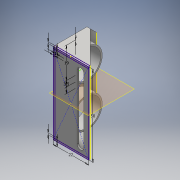
# Autodesk Inventor part: Ultra Sonic Sensor Mounting
Saved by Autodesk Inventor 2016 (Build 200138000, 138)
## iProperties
Created: 2016-05-08
Part Number: Ultra Sonic Sensor Mounting
Material: Generic
Document SubType Name: Modeling
Designer: Kenneth Daniel
Density: 1 g/cm^3
Appearance: Default
Author: Kenneth Daniel
Autodesk Inventor part; units mm, degrees
ref_plane "YZ Plane" through (0, 0, 0) normal (1, 0, 0) x (0, 1, 0)
ref_plane "XZ Plane" through (0, 0, 0) normal (0, 1, 0) x (-1, 0, 0)
ref_plane "XY Plane" through (0, 0, 0) normal (0, 0, 1) x (1, 0, 0)
sketch "Sketch1" plane through (0, 0, 0) normal (0, 1, 0) x (-1, 0, 0)
  line L0 (-11, 25) -> (-11, -25)
  line L1 (-11, -25) -> (11, -25)
  line L2 (11, -25) -> (11, 25)
  line L3 (11, 25) -> (-11, 25)
  line L4 (-11, 25) -> (11, -25) construction
  line L5 (-11, -25) -> (11, 25) construction
  line L6 (11, 25) -> (10, 25)
  line L7 (10, 25) -> (10, -25)
  line L8 (11, 25) -> (11, 24)
  line L9 (11, 24) -> (-11, 24)
  line L10 (11, -25) -> (11, -24)
  line L11 (11, -24) -> (-11, -24)
  point P0 (0, 0)
  dimension "d0" = 50
  dimension "d1" = 22
  dimension "d2" = 1
  dimension "d3" = 1
  dimension "d4" = 1
  constraints: 24 end point, 6 point on line, 4 perpendicular, 2 midpoint, 2 parallel, 1 vertical
  measures "d0" distance of L0.start L0.end
  measures "d1" distance of L1.end L0.end
  measures "d2" distance of L2.end L6.end
  measures "d3" distance of L2.end L8.end
  measures "d4" distance of L1.end L10.end
extrude "Extrusion1" add sketch "Sketch1" along normal blind 1
sketch "Sketch2" plane through (0, 1, 0) normal (0, 1, 0) x (1, 0, 0)
  line L0 (11, -25) -> (11, 25) projected
  line L1 (-11, -25) -> (11, -25) projected
  line L2 (11, -25) -> (-11, -25)
  line L3 (-11, -25) -> (-11, -24)
  line L4 (-11, 25) -> (-11, -25) projected
  line L5 (-11, -24) -> (11, -24)
  line L6 (-11, -25) -> (-10, -25)
  line L7 (-10, -25) -> (-10, 25)
  line L8 (11, 25) -> (-11, 25) projected
  line L9 (-11, 25) -> (-11, 24)
  line L10 (-11, 24) -> (11, 24)
  point P0 (0, 0)
  dimension "d7" = 1
  dimension "d8" = 1
  dimension "d9" = 1
  constraints: 14 end point, 6 point on line, 3 perpendicular, 1 collinear
  measures "d7" distance of L1.start L3.end
  measures "d8" distance of L1.start L6.end
  measures "d9" distance of L4.start L9.end
extrude "Extrusion2" add sketch "Sketch2" along normal blind 25 contours L1 L3 L5 L7 | L5 L4 L10 L7 | L10 L4 L8 L7
extrude "Extrusion3" add sketch "Sketch2" along normal blind 25 contours L1 L7 L5 L0 | L1 L3 L5 L7 | L10 L7 L8 L0 | L10 L4 L8 L7
sketch "Sketch3" plane through (-11, 0, 25) normal (0, 0, 1) x (1, 0, 0)
  point P0 (11, 0)
sketch "Sketch4" plane through (-11, 0, -25) normal (-1, 0, 0) x (0, 0, 1)
  line L0 (49, 26) -> (1, 26) projected
  line L1 (25, 26) -> (45, 26)
  line L2 (25, 26) -> (5, 26)
  line L3 (50, 0) -> (50, 26) projected
  line L4 (50, 26) -> (50, 21)
  line L5 (50, 21) -> (45, 26)
  line L6 (0, 0) -> (0, 26) projected
  line L7 (0, 26) -> (0, 21)
  line L8 (0, 21) -> (5, 26)
  line L9 (50, 26) -> (45, 26)
  line L10 (0, 26) -> (5, 26)
  line L11 (0, 26) -> (50, 26) projected
  point P0 (25, 0)
  dimension "d14" = 20
  dimension "d15" = 20
  dimension "d16" = 5
  dimension "d17" = 5
  constraints: 16 end point, 4 point on line, 2 collinear, 1 midpoint
  measures "d14" distance of L1.start L1.end
  measures "d15" distance of L1.start L2.end
  measures "d16" distance of L3.end L4.end
  measures "d17" distance of L6.end L7.end
extrude "Extrusion4" cut sketch "Sketch4" against normal blind 25
sketch "Sketch5" plane through (-11, 0, 25) normal (0, 0, 1) x (1, 0, 0)
  line L0 (1, 22) -> (1, 26) projected
  line L1 (1, 22) -> (22, 1)
  line L2 (22, 22) -> (1, 22) projected
  line L3 (1, 22) -> (22, 22)
  line L4 (22, 22) -> (22, 1)
  point P0 (11, 0)
  constraints: 6 end point, 1 collinear, 1 perpendicular
extrude "Extrusion5" cut sketch "Sketch5" against normal through all
sketch "Sketch6" plane through (-10, 1, 24) normal (1, 0, 0) x (0, 0, -1)
  line L0 (4, 25) -> (44, 25) projected
  line L1 (24, 25) -> (24, -1) construction
  line L2 (0, 21) -> (0, 0) construction
  line L3 (0, 12) -> (48, 12) construction
  line L4 (48, 0) -> (48, 21) construction
  line L5 (24, 12) -> (20.5, 12) construction
  line L6 (20.5, 12) -> (27.5, 12) construction
  line L7 (20.5, 12) -> (1.5, 12) construction
  circle A0 centre (11, 12) radius 9.5
  circle A1 centre (11, 12) radius 8.5
  dimension "d22" = 3.5
  dimension "d23" = 7
  dimension "d24" = 19
  dimension "d25" = 1
  constraints: 10 end point, 5 point on line, 3 midpoint, 1 centre point, 1 horizontal, 1 horizontal alignment, 1 vertical, 2 other
  measures "d22" distance of L5.start L5.end
  measures "d23" distance of L5.end L6.end
  measures "d24" distance of L5.end L7.end
extrude "Extrusion6" add sketch "Sketch6" along normal blind 7
extrude "Extrusion7" cut sketch "Sketch6" against normal blind 7 contours A1
ref_plane "Work Plane1" through (-11, 0, 0) normal (0, 0, 1) x (1, 0, 0)
mirror "Mirror1" about plane through (-11, 0, 0) normal (0, 0, 1) of "Extrusion6"
mirror "Mirror2" about plane through (-11, 0, 0) normal (0, 0, 1) of "Extrusion6"
sketch "Sketch7" plane through (-10, 13, -13) normal (1, 0, 0) x (0, 0, -1)
  circle A0 centre (0, 0) radius 8.5 projected
  point P0 (-13, -13)
extrude "Extrusion8" cut sketch "Sketch7" against normal blind 7
sketch "Sketch8" plane through (0, 1, 0) normal (0, 1, 0) x (1, 0, 0)
  line L0 (-10, -24) -> (11, -24) projected
  line L1 (11, -24) -> (6, -24)
  line L2 (6, -24) -> (6, -20) construction
  line L3 (11, 24) -> (-10, 24) construction
  line L4 (11, 24) -> (6, 24) construction
  line L5 (6, 24) -> (6, 20) construction
  line L6 (6, 20) -> (6, -20) construction
  line L7 (8.0416, 20) -> (8.0416, -20)
  line L8 (3.9584, -20) -> (3.9584, 20)
  arc A0 (8.0416, 20) -> (3.9584, 20) centre (6, 20) ccw
  arc A1 (3.9584, -20) -> (8.0416, -20) centre (6, -20) ccw
  point P0 (0, 0)
  point P1 (6, 0)
  dimension "d32" = 5
  dimension "d33" = 4
  dimension "d34" = 5
  dimension "d35" = 4
  constraints: 16 end point, 4 point on circle, 4 tangent, 2 centre point, 2 perpendicular, 2 point on line, 1 midpoint, 1 parallel, 1 vertical
  measures "d32" distance of L0.end L1.end
  measures "d33" distance of L1.end L2.end
  measures "d34" distance of L3.start L4.end
  measures "d35" distance of L4.end L5.end
extrude "Extrusion9" cut sketch "Sketch8" against normal blind 7
body "Solid1"
